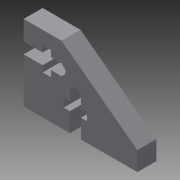
# Autodesk Inventor part: cornerBraceV01
Saved by Autodesk Inventor 2013 (Build 170138000, 138)
## iProperties
Created: 2014-06-26
Part Number: cornerBraceV01
Material: Generic
Document SubType Name: Modeling
Designer: Nano
Density: 1 g/cm^3
Author: Nano
Autodesk Inventor part; units mm, degrees
ref_plane "YZ Plane" through (0, 0, 0) normal (1, 0, 0) x (0, 1, 0)
ref_plane "XZ Plane" through (0, 0, 0) normal (0, 1, 0) x (-1, 0, 0)
ref_plane "XY Plane" through (0, 0, 0) normal (0, 0, 1) x (1, 0, 0)
sketch "Sketch1" plane through (0, 0, 0) normal (0, 0, 1) x (1, 0, 0)
  line L0 (0, 0) -> (38.1, 0)
  line L1 (38.1, 0) -> (38.1, 6.35)
  line L2 (12.7, 25.4) -> (0, 25.4)
  line L3 (0, 25.4) -> (0, 0)
  line L4 (12.7, 25.4) -> (38.1, 6.35)
  dimension "d2" = 6.35
  dimension "d3" = 12.7
  dimension "d4" = 25.4
  dimension "d5" = 38.1
  dimension "d7" = 27.94
  dimension "d8" = 38.1
  constraints: 10 end point, 2 parallel, 1 horizontal, 1 perpendicular
  measures "d2" distance of L1.end L0.end
  measures "d3" distance of L2.start L2.end
  measures "d4" distance of L2.end L0.start
  measures "d5" distance of L0.start L0.end
  measures "d7" distance from line of point (0, 0) L4
  measures "d8" distance from line of point (0, 0) L1
extrude "Extrusion1" add sketch "Sketch1" along normal blind 6.35
sketch "Sketch2" plane through (0, 0, 6.35) normal (0, 0, 1) x (1, 0, 0)
  line L0 (0, 0) -> (38.1, 0) projected
  line L1 (0, 25.4) -> (0, 0) projected
  line L2 (0, 18.8338) -> (-6.35, 18.8338)
  line L3 (0, 15.1254) -> (-6.35, 15.1254)
  line L4 (15.4827, -6.35) -> (15.4827, 0)
  line L5 (19.1911, -6.35) -> (19.1911, 0)
  line L6 (0, 18.8338) -> (12.7, 18.8338)
  line L7 (13.97, 17.5638) -> (13.97, 16.3954)
  line L8 (12.7, 15.1254) -> (0, 15.1254)
  line L9 (0, 15.1254) -> (0, 18.8338)
  line L10 (19.1911, 0) -> (15.4827, 0)
  line L11 (15.4827, 0) -> (15.4827, 12.7)
  line L12 (16.7527, 13.97) -> (17.9211, 13.97)
  line L13 (19.1911, 12.7) -> (19.1911, 0)
  line L14 (12.7, 18.8338) -> (13.97, 17.5638)
  line L15 (13.97, 16.3954) -> (12.7, 15.1254)
  line L16 (15.4827, 12.7) -> (16.7527, 13.97)
  line L17 (17.9211, 13.97) -> (19.1911, 12.7)
  line L18 (9.144, 20.9166) -> (6.35, 20.9166)
  line L19 (6.35, 20.9166) -> (6.35, 13.0426)
  line L20 (6.35, 13.0426) -> (9.144, 13.0426)
  line L21 (9.144, 13.0426) -> (9.144, 20.9166)
  line L22 (21.2739, 6.35) -> (13.3999, 6.35)
  line L23 (13.3999, 6.35) -> (13.3999, 9.144)
  line L24 (13.3999, 9.144) -> (21.2739, 9.144)
  line L25 (21.2739, 9.144) -> (21.2739, 6.35)
  point P0 (13.97, 15.1254)
  point P1 (13.97, 18.8338)
  point P2 (15.4827, 13.97)
  point P3 (19.1911, 13.97)
  point P4 (19.05, 0)
  dimension "d11" = 13.97
  dimension "d12" = 13.97
  dimension "d13" = 1.27
  dimension "d14" = 1.27
  dimension "d15" = 1.27
  dimension "d16" = 1.27
  dimension "d17" = 1.27
  dimension "d18" = 1.27
  dimension "d19" = 1.27
  dimension "d20" = 1.27
  dimension "d21" = 2.794
  dimension "d22" = 7.874
  dimension "d23" = 6.35
  dimension "d26" = 2.0828
  dimension "d27" = 2.0828
  dimension "d28" = 7.874
  dimension "d29" = 2.794
  dimension "d30" = 2.0828
  dimension "d31" = 6.35
  constraints: 48 end point, 10 point on line, 8 parallel, 6 horizontal, 4 collinear, 4 perpendicular, 2 vertical, 1 midpoint, 8 other
  measures "d11" distance of point (13.97, 15.125) L8.end
  measures "d12" distance of L10.end point (15.483, 13.97)
  measures "d13" distance of L6.end point (13.97, 18.834)
  measures "d14" distance of L7.start point (13.97, 18.834)
  measures "d15" distance of L7.end point (13.97, 15.125)
  measures "d16" distance of L8.start point (13.97, 15.125)
  measures "d17" distance of L11.end point (15.483, 13.97)
  measures "d18" distance of L12.start point (15.483, 13.97)
  measures "d19" distance of L12.end point (19.191, 13.97)
  measures "d20" distance of L13.start point (19.191, 13.97)
  measures "d21" distance of L20.end L19.end
  measures "d22" distance of L19.end L18.end
  measures "d23" distance between parallel lines of L1 L19
  measures "d26" distance between parallel lines of L6 L18
  measures "d27" distance between parallel lines of L20 L8
  measures "d28" distance of L23.end L24.end
  measures "d29" distance of L22.end L23.end
  measures "d30" distance between parallel lines of L25 L13
  measures "d31" distance between parallel lines of L10 L22
extrude "Extrusion2" cut sketch "Sketch2" against normal through all
equation "\"d14\" = d13"
equation "\"d15\" = d13"
equation "\"d16\" = d15"
equation "\"d17\" = d13"
equation "\"d18\" = d17"
equation "\"d19\" = d13"
equation "\"d20\" = d19"
equation "\"d26\" = d27"
equation "\"d30\" = d27"
equation "\"d31\" = d23"
body "Solid1"
